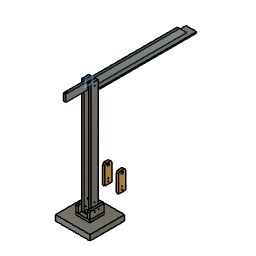
Kran v6 (Autodesk Fusion 360 design; units mm, degrees)
Autodesk Fusion 360 part; units mm, degrees
note: some values were not read from the file. Chosen so that the rebuilt part matches the saved one: which bodies a step acts on.
sketch "Skizze1" plane through (0, 0, 0) normal (0, 0, 1) x (1, 0, 0) in component "Turmaufnahme"
  line L0 (24, 25) -> (-24, 25)
  line L1 (-24, 25) -> (-24, -25)
  line L2 (-24, -25) -> (24, -25)
  line L3 (24, -25) -> (24, 25)
  line L4 (24, 25) -> (-24, -25) construction
  line L5 (-24, 25) -> (24, -25) construction
  dimension "d1" = 48
  dimension "d2" = 50
  constraint horizontal L0
  constraint perpendicular L0 L1
  constraint parallel L0 L2
  constraint parallel L1 L3
  constraint coincident L4 origin
  constraint coincident L5 origin
  measures "d1" distance of L1.end L2.end
  measures "d2" distance of L0.end L1.end
extrude "Extrusion1" add sketch "Skizze1" along normal blind 8 makes body 1 in component "Turmaufnahme"
sketch "Skizze3" plane through (0, 0, 8) normal (0, 0, 1) x (-1, 0, 0) in component "Turmaufnahme"
  line L0 (-24, 25) -> (-24, -25)
  line L1 (-24, -25) -> (24, -25)
  line L2 (24, -25) -> (24, 25)
  line L3 (24, 25) -> (-24, 25)
  line L4 (24, -25) -> (16, -25)
  line L5 (16, -25) -> (16, 25)
  line L6 (16, 25) -> (24, 25)
  line L7 (24, 25) -> (24, -25)
  dimension "d5" = 8
  constraint horizontal L4
  constraint vertical L5
  constraint horizontal L6
  constraint vertical L7
  constraint coincident L1.end L2.start
  measures "d5" distance of L1.end L4.end
extrude "Extrusion2" add sketch "Skizze3" along normal blind 25 separate body contours L1 L2 L3 L4 L5 L6 L7 makes body 2 in component "Turmaufnahme"
sketch "Skizze4" plane through (-16, 0, 0) normal (1, 0, 0) x (0, 1, 0) in component "Turmaufnahme"
  line L0 (25, 8) -> (25, 33)
  line L1 (25, 33) -> (-25, 33)
  line L2 (-25, 33) -> (-25, 8)
  circle A0 centre (-7, 25) radius 2
  circle A1 centre (7, 25) radius 2
  line L3 (-25, 8) -> (25, 8)
  dimension "d8" = 4
  dimension "d9" = 18
  dimension "d10" = 4
  dimension "d11" = 14
  dimension "d12" = 8
  dimension "d13" = 8
  measures "d8" diameter of A0
  measures "d9" distance of L2 A0.centre
  measures "d10" diameter of A1
  measures "d11" distance of A0.centre A1.centre
  measures "d12" distance of L1 A0.centre
  measures "d13" distance of L1 A1.centre
extrude "Extrusion3" cut sketch "Skizze4" against normal blind 8 contours A0 | A1 bodies 1 2 in component "Turmaufnahme"
sketch "Skizze5" plane through (0, 0, 8) normal (0, 0, 1) x (-1, 0, 0) in component "Turmaufnahme"
  line L0 (24, 25) -> (-24, 25)
  line L1 (-24, 25) -> (-24, -25)
  line L2 (-24, -25) -> (24, -25)
  line L3 (-8, -12.5) -> (8, -12.5)
  line L4 (8, -12.5) -> (8, 12.5)
  line L5 (8, 12.5) -> (-8, 12.5)
  line L6 (-8, 12.5) -> (-8, -12.5)
  line L7 (-8, -12.5) -> (8, 12.5) construction
  line L8 (8, -12.5) -> (-8, 12.5) construction
  line L9 (24, -25) -> (24, 25)
  dimension "d16" = 16
  dimension "d17" = 25
  constraint horizontal L3
  constraint perpendicular L3 L4
  constraint parallel L3 L5
  constraint parallel L4 L6
  constraint coincident L7 origin
  constraint coincident L8 origin
  measures "d16" distance of L4.end L5.end
  measures "d17" distance of L3.end L4.end
extrude "Extrusion4" add sketch "Skizze5" along normal blind 4 separate body contours L3 L4 L5 L6 makes body 3 in component "Turmaufnahme"
sketch "Skizze6" plane through (0, 0, 12) normal (0, 0, 1) x (-1, 0, 0) in component "Turmaufnahme"
  line L0 (-8, 12.5) -> (-8, -12.5)
  line L1 (-8, -12.5) -> (8, -12.5)
  line L2 (8, -12.5) -> (8, 12.5)
  line L3 (8, 12.5) -> (-8, 12.5)
  circle A0 centre (0, 0) radius 2
  dimension "d20" = 4
  constraint coincident A0.centre origin
  measures "d20" diameter of A0
extrude "Extrusion5" cut sketch "Skizze6" against normal blind 24 contours A0 bodies 1 3 in component "Turmaufnahme"
chamfer "Fase1" distance 5 angle 45 1 edges at (-20, -25, 33) on bodies 2 in component "Turmaufnahme"
mirror "Spiegeln1" about plane through (0, 0, 0) normal (1, 0, 0) of bodies 2 makes body 4 in component "Turmaufnahme"
sketch "Skizze2" plane through (0, 0, 0) normal (0, 0, -1) x (1, 0, 0) in component "Grundplate"
  circle A0 centre (0, 0) radius 2
  line L0 (24, -25) -> (24, 25)
  line L1 (24, 25) -> (-24, 25)
  line L2 (-24, 25) -> (-24, -25)
  line L3 (-24, -25) -> (24, -25)
  line L4 (60, 60) -> (-60, 60)
  line L5 (-60, 60) -> (-60, -60)
  line L6 (-60, -60) -> (60, -60)
  line L7 (60, -60) -> (60, 60)
  line L8 (60, 60) -> (-60, -60) construction
  line L9 (-60, 60) -> (60, -60) construction
  dimension "d35" = 120
  dimension "d36" = 120
  constraint horizontal L4
  constraint perpendicular L4 L5
  constraint parallel L4 L6
  constraint parallel L5 L7
  constraint coincident L8 A0.centre
  constraint coincident L9 A0.centre
  constraint coincident A0.centre origin
  measures "d35" distance of L5.end L6.end
  measures "d36" distance of L4.end L5.end
extrude "Extrusion3'" add sketch "Skizze2" along normal blind 19 separate body contours L0 L1 L2 L3 | L4 L5 L6 L7 makes body 5 in component "Grundplate"
sketch "Skizze3 (2)" plane through (0, 0, -19) normal (0, 0, -1) x (1, 0, 0) in component "Grundplate"
  circle A0 centre (0, 0) radius 2
  line L0 (60, -60) -> (60, 60)
  line L1 (60, 60) -> (-60, 60)
  line L2 (-60, 60) -> (-60, -60)
  line L3 (-60, -60) -> (60, -60)
  circle A1 centre (0, 0) radius 5
  dimension "d39" = 10
  constraint coincident A0.centre A1.centre
  measures "d39" diameter of A1
extrude "Extrusion4'" cut sketch "Skizze3 (2)" against normal blind 4 contours A1 bodies 5 in component "Grundplate"
sketch "Skizze2 (2)" plane through (-16, 0, 0) normal (1, 0, 0) x (0, 1, 0) in component "Turmhälfte limks"
  line L0 (-20, 33) -> (-25, 28)
  line L1 (-25, 28) -> (-25, 8)
  line L2 (-25, 8) -> (25, 8)
  line L3 (25, 8) -> (25, 33)
  line L4 (25, 33) -> (-20, 33)
  circle A0 centre (7, 25) radius 2
  circle A1 centre (-7, 25) radius 2
  line L5 (-12.5, 408) -> (12.5, 408)
  line L6 (12.5, 408) -> (12.5, 8)
  line L7 (12.5, 8) -> (-12.5, 8)
  line L8 (-12.5, 8) -> (-12.5, 408)
  circle A2 centre (-7, 25) radius 2
  circle A3 centre (7, 25) radius 2
  dimension "d44" = 25
  dimension "d45" = 400
  dimension "d46" = 12.5
  constraint horizontal L5
  constraint vertical L6
  constraint horizontal L7
  constraint vertical L8
  constraint collinear L2 L7
  measures "d44" distance of L5.start L5.end
  measures "d45" distance of L5.start L7.end
  measures "d46" distance of L3 L6
extrude "Extrusion1'" add sketch "Skizze2 (2)" along normal blind 8 separate body contours L4 L5 L6 L8 | L2 L4 L6 L7 L8 makes body 6 in component "Turmhälfte limks"
sketch "Skizze3 (3)" plane through (-8, 0, 0) normal (1, 0, 0) x (0, 1, 0) in component "Turmhälfte limks"
  circle A0 centre (-7, 25) radius 2
  circle A1 centre (7, 25) radius 2
  line L0 (-12.5, 8) -> (12.5, 8)
  line L1 (12.5, 8) -> (12.5, 408)
  line L2 (12.5, 408) -> (-12.5, 408)
  line L3 (-12.5, 408) -> (-12.5, 8)
  line L4 (-12.5, 408) -> (12.5, 408)
  line L5 (12.5, 408) -> (12.5, 388)
  line L6 (12.5, 388) -> (-12.5, 388)
  line L7 (-12.5, 388) -> (-12.5, 408)
  dimension "d49" = 20
  constraint horizontal L4
  constraint vertical L5
  constraint horizontal L6
  constraint vertical L7
  constraint coincident L2.end L3.start
  measures "d49" distance of L2.end L6.end
sketch "Skizze5 (2)" plane through (-8, 0, 0) normal (1, 0, 0) x (0, 1, 0) in component "Turmhälfte limks"
  circle A0 centre (-7, 25) radius 2
  circle A1 centre (7, 25) radius 2
  line L0 (-12.5, 8) -> (12.5, 8)
  line L1 (12.5, 8) -> (12.5, 408)
  line L2 (12.5, 408) -> (-12.5, 408)
  line L3 (-12.5, 408) -> (-12.5, 8)
  line L4 (0, 8) -> (0, 408) construction
  circle A2 centre (0, 396) radius 2
  circle A3 centre (0, 45) radius 2
  dimension "d63" = 4
  dimension "d64" = 12
  dimension "d65" = 4
  dimension "d66" = 37
  constraint midpoint L0 L4.start
  constraint midpoint L2 L4.end
  constraint coincident L4 A2.centre
  constraint coincident L4 A3.centre
  measures "d63" diameter of A2
  measures "d64" distance of L4.end A2.centre
  measures "d65" diameter of A3
  measures "d66" distance of L4.start A3.centre
extrude "Extrusion5'" cut sketch "Skizze5 (2)" against normal blind 8 contours A2 | A3 bodies 6 in component "Turmhälfte limks"
sketch "Skizze6 (2)" plane through (-8, 0, 0) normal (1, 0, 0) x (0, 1, 0) in component "Turmhälfte limks"
  circle A0 centre (0, 45) radius 2
  circle A1 centre (0, 396) radius 2
  circle A2 centre (-7, 25) radius 2
  circle A3 centre (7, 25) radius 2
  line L0 (-12.5, 8) -> (12.5, 8)
  line L1 (12.5, 8) -> (12.5, 408)
  line L2 (12.5, 408) -> (-12.5, 408)
  line L3 (-12.5, 408) -> (-12.5, 8)
  line L4 (-12.5, 408) -> (12.5, 408)
  line L5 (12.5, 408) -> (12.5, 388)
  line L6 (12.5, 388) -> (-12.5, 388)
  line L7 (-12.5, 388) -> (-12.5, 408)
  dimension "d69" = 20
  constraint horizontal L4
  constraint vertical L5
  constraint horizontal L6
  constraint vertical L7
  constraint coincident L2.end L3.start
  measures "d69" distance of L2.end L6.end
mirror "Komponente spiegeln1" about plane through (0, 0, 0) normal (0, 0, 1) of bodies 6 makes body 7 in component "Turmhälfte rechts"
sketch "Skizze1 (2)" plane through (16, 0, 0) normal (1, 0, 0) x (0, 1, 0)
  circle A0 centre (0, 45) radius 2
  circle A1 centre (0, 396) radius 2
  circle A2 centre (-7, 25) radius 2
  circle A3 centre (7, 25) radius 2
  line L0 (-12.5, 8) -> (12.5, 8)
  line L1 (12.5, 8) -> (12.5, 408)
  line L2 (12.5, 408) -> (-12.5, 408)
  line L3 (-12.5, 408) -> (-12.5, 8)
extrude "Extrusion1''" cut sketch "Skizze1 (2)" along normal blind 12 contours A1 sketch seen with x (-1, 0, 0) y (0, 1, 0) z (0, 0, -1) at (0, 0, 0) in component "Turmhälfte rechts"
sketch "Skizze2 (3)" plane through (-4, 0, 0) normal (1, 0, 0) x (0, 1, 0)
  circle A0 centre (0, 396) radius 2
  line L0 (-12.5, 388) -> (12.5, 388)
  line L1 (12.5, 388) -> (12.5, 408)
  line L2 (12.5, 408) -> (-12.5, 408)
  line L3 (-12.5, 408) -> (-12.5, 388)
sketch "Skizze7" plane through (-4, 0, 0) normal (1, 0, 0) x (0, 1, 0) in component "Turmhälfte limks"
  line L0 (-12.4558, 407.9704) -> (12.5442, 407.9704)
  line L1 (12.5442, 407.9704) -> (12.5442, 387.9704)
  line L2 (12.5442, 387.9704) -> (-12.4558, 387.9704)
  line L3 (-12.4558, 387.9704) -> (-12.4558, 407.9704)
  dimension "d82" = 25
  dimension "d83" = 20
  constraint horizontal L0
  constraint vertical L1
  constraint horizontal L2
  constraint vertical L3
  measures "d82" distance of L0.start L0.end
  measures "d83" distance of L0.start L2.end
extrude "Extrusion7" add sketch "Skizze2 (3)" against normal blind 4 separate body contours A0 | L0 L1 L2 L3 makes body 8 in component "Turmhälfte limks"
sketch "Skizze3 (4)" plane through (-4, 0, 0) normal (1, 0, 0) x (0, 1, 0)
  circle A0 centre (0, 396) radius 2
extrude "Extrusion8" cut sketch "Skizze3 (4)" against normal blind 4 bodies 8 in component "Turmhälfte limks"
mirror "Komponente spiegeln2" about plane through (0, 0, 0) normal (0, 0, 1) of bodies 6 8 makes body 9 at (-16, 2.0782, -13.0507) makes body 10 at (-4, -0.0498, -404.6648) in component "Turmhälfte rechts (1)"
sketch "Skizze5 (3)" plane through (-4, 0, 0) normal (1, 0, 0) x (0, 1, 0) in component "Ausleger"
  line L0 (-88, 408.5) -> (332, 408.5)
  line L1 (332, 408.5) -> (332, 383.5)
  line L2 (332, 383.5) -> (-88, 383.5)
  line L3 (-88, 383.5) -> (-88, 408.5)
  circle A0 centre (0, 396) radius 2
  circle A1 centre (0, 396) radius 2
  dimension "d88" = 420
  dimension "d89" = 25
  dimension "d90" = 4
  dimension "d91" = 12.5
  dimension "d92" = 88
  constraint horizontal L0
  constraint vertical L1
  constraint horizontal L2
  constraint vertical L3
  constraint concentric A0 A1
  measures "d88" distance of L0.start L0.end
  measures "d89" distance of L0.start L2.end
  measures "d90" diameter of A0
  measures "d91" distance of L2 A0.centre
  measures "d92" distance of L3 A0.centre
extrude "Extrusion2'" add sketch "Skizze5 (3)" along normal blind 8 separate body makes body 11 in component "Ausleger"
chamfer "Fase2" distance 25 angle 45 1 edges at (0, 332, 408.5) on bodies 11 in component "Ausleger"
sketch "Skizze6 (3)" plane through (0, 0, 408.5) normal (0, 0, 1) x (-1, 0, 0) in component "Ausleger"
  line L0 (-4, -307) -> (4, -307)
  line L1 (4, -307) -> (4, 88)
  line L2 (4, 88) -> (-4, 88)
  line L3 (-4, 88) -> (-4, -307)
  line L4 (0, 88) -> (0, 72) construction
  circle A0 centre (0, 80) radius 1.5
  dimension "d98" = 3
  dimension "d99" = 8
  constraint midpoint L2 L4.start
  constraint perpendicular L2 L4
  constraint midpoint L4 A0.centre
  measures "d98" diameter of A0
  measures "d99" distance of L2 A0.centre
extrude "Extrusion3''" cut sketch "Skizze6 (3)" against normal blind 25 contours A0 bodies 11 in component "Ausleger"
sketch "Skizze7 (2)" plane through (0, 0, 383.5) normal (0, 0, -1) x (1, 0, 0) in component "Ausleger"
  circle A0 centre (0, 80) radius 1.5
  line L0 (-4, 88) -> (-4, -332)
  line L1 (-4, -332) -> (4, -332)
  line L2 (4, -332) -> (4, 88)
  line L3 (4, 88) -> (-4, 88)
  line L4 (-18.5, -15) -> (18.5, -15)
  line L5 (18.5, -15) -> (18.5, -352)
  line L6 (18.5, -352) -> (-18.5, -352)
  line L7 (-18.5, -352) -> (-18.5, -15)
  line L8 (0, -15) -> (0, 191) construction
  dimension "d102" = 37
  dimension "d103" = 337
  dimension "d104" = 103
  constraint horizontal L4
  constraint vertical L5
  constraint horizontal L6
  constraint vertical L7
  constraint midpoint L4 L8.start
  constraint perpendicular L4 L8
  constraint midpoint L3 L8
  measures "d102" distance of L4.start L4.end
  measures "d103" distance of L4.start L6.end
  measures "d104" distance of L3 L4
extrude "Extrusion4''" add sketch "Skizze7 (2)" along normal blind 4 separate body contours L0 L1 L2 L4 | L0 L1 L2 L4 L5 L6 L7 makes body 12 in component "Ausleger"
sketch "Skizze4 (2)" plane through (4, 0, 0) normal (1, 0, 0) x (0, 1, 0)
  line L0 (332, 383.5) -> (307, 408.5)
  line L1 (307, 408.5) -> (-88, 408.5)
  line L2 (-88, 408.5) -> (-88, 383.5)
  line L3 (-88, 383.5) -> (332, 383.5)
  circle A0 centre (0, 396) radius 2
sketch "Skizze5 (4)" plane through (0, 0, 379.5) normal (0, 0, -1) x (1, 0, 0)
  line L0 (-18.5, -352) -> (18.5, -352)
  line L1 (18.5, -352) -> (18.5, -15)
  line L2 (18.5, -15) -> (-18.5, -15)
  line L3 (-18.5, -15) -> (-18.5, -352)
sketch "Skizze1 (3)" plane through (0, 0, 0) normal (1, 0, 0) x (0, 1, 0) in component "Handantrieb"
  line L0 (50, 0) -> (116, 0)
  line L1 (116, 0) -> (116, 25)
  line L2 (116, 25) -> (50, 25)
  line L3 (50, 25) -> (50, 0)
  line L4 (50, 12.5) -> (116, 12.5)
  circle A0 centre (58, 12.5) radius 4
  circle A1 centre (108.5, 12.5) radius 2
  circle A2 centre (98.5, 12.5) radius 2
  dimension "d115_1" = 66
  dimension "d116_1" = 25
  dimension "d117_1" = 8
  dimension "d118_1" = 4
  dimension "d119_1" = 4
  dimension "d120_1" = 8
  dimension "d121_1" = 7.5
  dimension "d122_1" = 10
  constraint horizontal L0
  constraint vertical L1
  constraint horizontal L2
  constraint vertical L3
  constraint midpoint L3 L4.start
  constraint midpoint L1 L4.end
  constraint coincident L4 A0.centre
  constraint coincident L4 A1.centre
  constraint coincident L4 A2.centre
  measures "d115_1" distance of L0.start L0.end
  measures "d116_1" distance of L0.start L2.end
  measures "d117_1" diameter of A0
  measures "d118_1" diameter of A1
  measures "d119_1" diameter of A2
  measures "d120_1" distance of L4.start A0.centre
  measures "d121_1" distance of L4.end A1.centre
  measures "d122_1" distance of A1.centre A2.centre
extrude "Extrusion1'''" add sketch "Skizze1 (3)" along normal blind 8 separate body contours L0 L1 L3 L4 A0 A1 A2 | L1 L2 L3 L4 A0 A1 A2 makes body 13 in component "Handantrieb"
chamfer "Fase1'" distance 5 angle 45 1 edges at (4, 50, 25) on bodies 13 in component "Handantrieb"
chamfer "Fase2'" distance 5 angle 45 1 edges at (4, 50, 0) on bodies 13 in component "Handantrieb"
mirror "Komponente spiegeln3" about plane through (0, 0, 0) normal (0, 0, 1) of bodies 13 makes body 14 in component "Handantrieb(Spiegeln)"
component "Grundplate" placed x (1, 0, 0) y (0, 1, 0) z (0, 0, 1) at (0, 0, 0)
component "Turmhälfte limks" placed x (1, 0, 0) y (0, 1, 0) z (0, 0, 1) at (0, 0, 0)
component "Ausleger" placed x (1, 0, 0) y (0, 1, 0) z (0, 0, 1) at (0, 0, 0)
component "Turmaufnahme" placed x (1, 0, 0) y (0, 1, 0) z (0, 0, 1) at (0, 0, 0)
component "Turmhälfte rechts (1)" placed x (-1, 0, 0) y (0, 1, 0) z (0, 0, -1) at (0, 0, 0)
component "Handantrieb" placed x (1, 0, 0) y (0, 0, -1) z (0, 1, 0) at (20, 71.2686, 156.2686)
component "Handantrieb(Spiegeln)" placed x (-1, 0, 0) y (0, 0, -1) z (0, -1, 0) at (-20, 71.2686, 156.2686)
equation "d46 = ( 25 / 2 ) * 1 mm"
equation "d91 = ( 25 / 2 ) * 1 mm"
named bodies: "Horizontale Platte", "Plätchen", "Turmaufnahme links", "Turmaufnahme rechts", "Seite"
